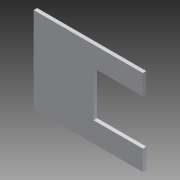
# Autodesk Inventor part: mixer support
Saved by Autodesk Inventor 2011 (Build 150239000, 239)
## iProperties
Created: 2013-11-09
Part Number: mixer support
Document SubType Name: Modeling
Designer: Devon
Density: 1 g/cm^3
Author: Devon
Autodesk Inventor part; units mm, degrees
ref_plane "YZ Plane" through (0, 0, 0) normal (1, 0, 0) x (0, 1, 0)
ref_plane "XZ Plane" through (0, 0, 0) normal (0, 1, 0) x (-1, 0, 0)
ref_plane "XY Plane" through (0, 0, 0) normal (0, 0, 1) x (1, 0, 0)
sketch "Sketch1" plane through (0, 0, 0) normal (0, 0, 1) x (1, 0, 0)
  line L0 (0, 0) -> (196.088, 0)
  line L1 (196.088, 153.9748) -> (0, 153.9748)
  line L2 (0, 153.9748) -> (0, 0)
  line L3 (119.888, 36.3474) -> (196.088, 36.3474)
  line L4 (119.888, 117.6274) -> (196.088, 117.6274)
  line L5 (196.088, 0) -> (196.088, 36.3474)
  line L6 (196.088, 117.6274) -> (196.088, 153.9748)
  line L7 (119.888, 117.6274) -> (107.5944, 117.6274)
  line L8 (119.888, 36.3474) -> (107.5944, 36.3474)
  line L9 (107.5944, 36.3474) -> (107.5944, 117.6274)
  dimension "d0" = 196.088
  dimension "d1" = 153.9748
  dimension "d7" = 12.2936
  dimension "d8" = 12.2936
  constraints: 20 end point, 7 perpendicular, 4 parallel, 1 horizontal
  measures "d0" distance of L1.end L1.start
  measures "d1" distance of L1.start L0.end
  measures "d7" distance of L4.start L7.end
  measures "d8" distance of L3.start L8.end
extrude "Extrusion1" add sketch "Sketch1" along normal blind 6.35
body "Solid1"
